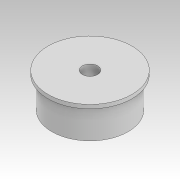
# Autodesk Inventor part: BearingAdapter
Saved by Autodesk Inventor 2020 (Build 240168000, 168)
## iProperties
Created: 2022-01-15
Part Number: BearingAdapter
Material: Generic
Document SubType Name: Modeling
Designer: DDeGo
Density: 1 g/cm^3
Appearance: Default
Author: DDeGo
Autodesk Inventor part; units mm, degrees
ref_plane "YZ Plane" through (0, 0, 0) normal (1, 0, 0) x (0, 1, 0)
ref_plane "XZ Plane" through (0, 0, 0) normal (0, 1, 0) x (-1, 0, 0)
ref_plane "XY Plane" through (0, 0, 0) normal (0, 0, 1) x (1, 0, 0)
sketch "Sketch1" plane through (0, 0, 0) normal (0, 0, 1) x (1, 0, 0)
  line L0 (0, 0) -> (5, 0)
  line L1 (5, 0) -> (5, 4)
  line L2 (5, 4) -> (5.5, 4)
  line L3 (5.5, 4) -> (5.5, 4.5)
  line L4 (5.5, 4.5) -> (1, 4.5)
  line L5 (1, 4.5) -> (1, 0.75)
  line L6 (1, 0.75) -> (0, 0.75)
  line L7 (0, 0.75) -> (0, 0)
  dimension "d0" = 1
  dimension "d1" = 4
  dimension "d2" = 0.5
  dimension "d3" = 0.5
  dimension "d4" = 5
  dimension "d5" = 0.75
  constraints: 16 end point, 7 perpendicular, 1 horizontal
  measures "d0" distance between parallel lines of L7 L5
  measures "d1" distance between parallel lines of L0 L2
  measures "d2" distance of L2.end L3.end
  measures "d3" distance of L1.end L2.end
  measures "d4" distance between parallel lines of L7 L1
  measures "d5" distance between parallel lines of L0 L6
revolve "Revolution1" add sketch "Sketch1" angle 360 about axis through (0, 0.75, 0) along (0, -1, 0)
body "Solid1"
